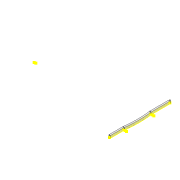
# Autodesk Inventor part: Part_3
Saved by Autodesk Inventor 2022 (Build 260153000, 153)
## iProperties
Created: 2022-04-26
Part Number: Part_3
Material: Generic
Document SubType Name: Modeling
Designer: dell
Density: 1 g/cm^3
Appearance: Default
Author: dell
Autodesk Inventor part; units mm, degrees
ref_plane "YZ Plane" through (0, 0, 0) normal (1, 0, 0) x (0, 1, 0)
ref_plane "XZ Plane" through (0, 0, 0) normal (0, 1, 0) x (-1, 0, 0)
ref_plane "XY Plane" through (0, 0, 0) normal (0, 0, 1) x (1, 0, 0)
sketch "Sketch1" plane through (0, 0, 0) normal (0, 1, 0) x (-1, 0, 0)
  line L0 (0, 0) -> (0, -233.87) construction
  line L1 (-3, 0) -> (-3, -233.87)
  line L2 (3, -233.87) -> (3, 0)
  arc A0 (3, 0) -> (-3, 0) centre (0, 0) ccw
  arc A1 (-3, -233.87) -> (3, -233.87) centre (0, -233.87) ccw
  circle A2 centre (0, 0) radius 1.5
  circle A3 centre (0, -233.87) radius 1.5
  circle A4 centre (0, -158.374) radius 1.5
  circle A5 centre (0, -53.738) radius 1.5
  arc A6 (3, -53.738) -> (3, -158.374) centre (399.5638, -106.056) ccw
  arc A7 (-3, -53.738) -> (-3, -158.374) centre (393.5638, -106.056) ccw
  point P0 (0, -116.935)
  dimension "d0" = 233.87
  dimension "d1" = 6
  dimension "d2" = 3
  dimension "d3" = 3
  dimension "d6" = 3
  dimension "d7" = 158.374
  dimension "d8" = 3
  dimension "d9" = 53.738
  dimension "d10" = 400
  dimension "d11" = 400
  constraints: 8 centre point, 8 end point, 8 point on circle, 6 point on line, 4 horizontal alignment, 4 tangent, 2 coincident, 1 midpoint, 1 parallel, 1 vertical
  measures "d0" distance of L0.start L0.end
  measures "d1" diameter of A1
  measures "d2" diameter of A2
  measures "d3" diameter of A3
  measures "d6" diameter of A4
  measures "d7" distance of L0.start A4.centre
  measures "d8" diameter of A5
  measures "d9" distance of L0.start A5.centre
  measures "d10" radius of A6
  measures "d11" radius of A7
extrude "Extrusion1" add sketch "Sketch1" along normal blind 8 contours A0 L2 A6 A1 L1 | L1 A7
fillet "Fillet1" radius 10 4 edges at (3, 4, -53.738) (3, 4, -158.374) (-3, 4, -158.374) (-3, 4, -53.738)
sketch "Sketch2" plane through (0, 0, 0) normal (0, -1, 0) x (1, 0, 0)
  arc A0 (-3, -53.0853) -> (-2.9162, -54.3772) centre (7, -53.0853) ccw projected
  arc A1 (-2.9162, -157.7348) -> (-2.9162, -54.3772) centre (-399.5638, -106.056) ccw projected
  arc A2 (-2.9162, -157.7348) -> (-3, -159.0267) centre (7, -159.0267) ccw projected
  line L0 (-3, -233.87) -> (-3, -159.0267) projected
  arc A3 (-3, -233.87) -> (3, -233.87) centre (0, -233.87) ccw projected
  line L1 (3, -159.0267) -> (3, -233.87) projected
  arc A4 (3.0838, -157.7348) -> (3, -159.0267) centre (13, -159.0267) ccw projected
  arc A5 (3.0838, -157.7348) -> (3.0838, -54.3772) centre (-393.5638, -106.056) ccw projected
  arc A6 (3, -53.0853) -> (3.0838, -54.3772) centre (13, -53.0853) ccw projected
  line L2 (3, 0) -> (3, -53.0853) projected
  arc A7 (3, 0) -> (-3, 0) centre (0, 0) ccw projected
  line L3 (-3, -53.0853) -> (-3, 0) projected
  circle A8 centre (0, 0) radius 1.5 projected
  circle A9 centre (0, -233.87) radius 1.5 projected
  circle A10 centre (0, -53.738) radius 1.5 projected
  circle A11 centre (0, -158.374) radius 1.5 projected
body "Solid1"
